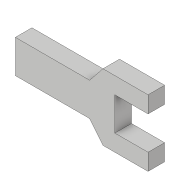
# Autodesk Inventor part: wrench
Saved by Autodesk Inventor 2019 (Build 230136000, 136)
## iProperties
Created: 2021-06-13
Part Number: wrench
Material: Generic
Document SubType Name: Modeling
Designer: dmulr
Density: 1 g/cm^3
Appearance: Default
Author: dmulr
Autodesk Inventor part; units mm, degrees
ref_plane "YZ Plane" through (0, 0, 0) normal (1, 0, 0) x (0, 1, 0)
ref_plane "XZ Plane" through (0, 0, 0) normal (0, 1, 0) x (-1, 0, 0)
ref_plane "XY Plane" through (0, 0, 0) normal (0, 0, 1) x (1, 0, 0)
sketch "Sketch2" plane through (0, 0, 0) normal (0, 0, 1) x (1, 0, 0)
  line L0 (500, -250) -> (160, -250)
  line L1 (-500, -125) -> (-500, 125)
  line L2 (160, 250) -> (500, 250)
  line L3 (500, -250) -> (-500, 250) construction
  line L4 (-500, -250) -> (500, 250) construction
  line L5 (250, 125) -> (250, -125)
  line L6 (500, 250) -> (500, 125)
  line L7 (500, -125) -> (500, -250)
  line L8 (-500, 125) -> (60, 125)
  line L9 (250, 125) -> (500, 125)
  line L10 (-500, -125) -> (60, -125)
  line L11 (250, -125) -> (500, -125)
  line L12 (160, 250) -> (60, 125)
  line L13 (160, -250) -> (60, -125)
  point P0 (0, 0)
  dimension "d0" = 1000
  dimension "d1" = 500
  dimension "d2" = 1000
  constraints: 28 end point, 11 perpendicular, 3 parallel, 2 midpoint, 1 horizontal
  measures "d0" distance of L3.end L2.end
  measures "d1" distance of L4.start L3.end
  measures "d2" distance of L1.start L7.start
extrude "Extrusion1" add sketch "Sketch2" along normal blind 125
body "Solid1"
